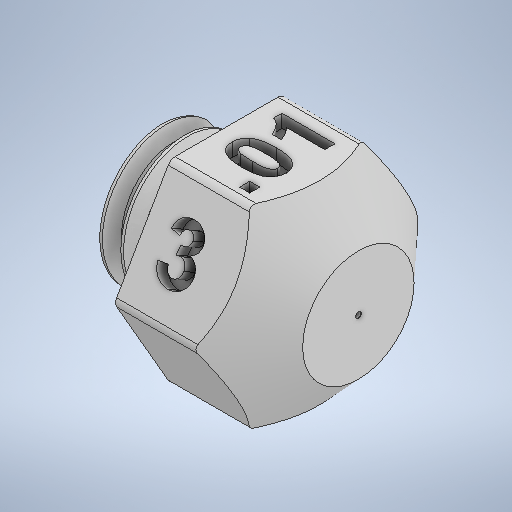
# Autodesk Inventor part: Part1
Saved by Autodesk Inventor 2025.2 (Build 292293000, 293)
## iProperties
Created: 2026-03-09
Part Number: Part1
Material: Generic
Document SubType Name: Modeling
Designer: Simon
Density: 1 g/cm^3
Appearance: Default
Author: Simon
Autodesk Inventor part; units mm, degrees
ref_plane "YZ Plane" through (0, 0, 0) normal (1, 0, 0) x (0, 1, 0)
ref_plane "XZ Plane" through (0, 0, 0) normal (0, 1, 0) x (-1, 0, 0)
ref_plane "XY Plane" through (0, 0, 0) normal (0, 0, 1) x (1, 0, 0)
sketch "Sketch1" plane through (0, 0, 0) normal (0, 0, 1) x (1, 0, 0)
  line L0 (0, 0) -> (0, 1.25)
  line L1 (0, 1.25) -> (50, 1.25)
  line L2 (0, 0) -> (0, 0.1062)
  line L3 (0, 0.1062) -> (50, 0.1062)
  line L4 (0, 0) -> (0, 0.1111)
  line L5 (0, 0.1111) -> (50, 0.1111)
  line L6 (0, 0) -> (0, 2.5)
  line L7 (0, 2.5) -> (2.5, 2.5)
  line L8 (2.5, 2.5) -> (2.5, 1.25)
  line L9 (2.5, 1.25) -> (2.5, 4.25)
  line L10 (2.5, 1.25) -> (6.7109, 1.25) construction
  line L11 (2.5, 4.25) -> (5.5, 4.25)
  line L12 (5.5, 4.25) -> (5.5, 1.25)
  line L13 (5.5, 1.25) -> (7.4811, 0.1062)
  line L14 (5.5, 1.25) -> (9.25, 1.25) construction
  line L15 (7.4811, 0.1062) -> (7.4992, 0.1111)
  line L16 (7.4811, 0.1062) -> (7.4998, 0.1062) construction
  line L17 (7.4992, 0.1111) -> (7.4992, 2.1111)
  line L18 (7.4992, 2.1111) -> (5.5, 4.25)
  line L19 (0, 0) -> (50, 0)
  dimension "d0" = 1.25
  dimension "d1" = 50
  dimension "d2" = 0.1062
  dimension "d3" = 0.1111
  dimension "d4" = 2.5
  dimension "d5" = 2.5
  dimension "d6" = 3
  dimension "d8" = 3
  dimension "d9" = 30
  dimension "d10" = 15
  dimension "d12" = 2
  dimension "d13" = 50
  constraints: 40 end point, 7 perpendicular, 7 point on line, 5 horizontal, 2 vertical, 1 equal length
  measures "d0" distance of L0.start L0.end
  measures "d1" distance of L0.end L1.end
  measures "d2" distance of L0.start L2.end
  measures "d3" distance of L0.start L4.end
  measures "d4" distance of L0.start L6.end
  measures "d5" distance of L6.end L7.end
  measures "d6" distance of L8.end L9.end
  measures "d8" distance of L9.end L11.end
  measures "d9" angle of L13 L14
  measures "d10" angle of L16 L15
  measures "d12" distance of L15.end L17.end
  measures "d13" distance of L0.start L19.end
revolve "Revolution1" add sketch "Sketch1" angle 360 about axis through (0, 0, 0) along (1, 0, 0) contours L13 L5 L15 | L6 L7 L8 L1 | L13 L1 L17 L5 | L8 L9 L11 L12 L1 | L12 L18 L17 L1
sketch "Sketch2" plane through (2.5, 0, 0) normal (-1, 0, 0) x (0, 0, 1)
  circle A0 centre (0, 0) radius 4.25 projected
  line L0 (-4.25, 0) -> (4.25, 0)
  circle A1 centre (0, 0) radius 0.1062 projected
  line L1 (4.25, 0) -> (2.125, -3.6806)
  line L2 (2.125, -3.6806) -> (-2.125, -3.6806)
  line L3 (-2.125, -3.6806) -> (-4.25, 0)
  line L4 (-4.25, 0) -> (-2.125, 3.6806)
  line L5 (-2.125, 3.6806) -> (2.125, 3.6806)
  line L6 (2.125, 3.6806) -> (4.25, 0)
  circle A2 centre (0, 0) radius 1.25
  constraints: 14 end point, 2 coincident, 2 point on circle, 1 centre point, 1 horizontal, 13 other
extrude "Extrusion1" cut sketch "Sketch2" against normal through all contours L6 A0 | A0 L1 | L5 A0 | A0 L2 | L4 A0 | A0 L3
fillet "Fillet1" radius 0.3 6 edges at (4, 3.6806, 2.125) (4, 3.6806, -2.125) (4, 0, -4.25) (4, -3.6806, -2.125) (4, -3.6806, 2.125) (4, 0, 4.25)
sketch "Sketch3" plane through (0, 0, 0) normal (0, 0, 1) x (1, 0, 0)
  line L0 (-0.35, 1.8938) -> (0.45, 1.8938)
  line L1 (-0.35, 1.8938) -> (0.05, 2.5866)
  line L2 (-0.35, 1.8938) -> (0.45, 1.8938) construction
  line L3 (0.05, 2.5866) -> (0.45, 1.8938)
  line L4 (-0.0972, 3.8266) -> (0.7028, 3.8266) construction
  line L5 (0.05, 2.5866) -> (0.05, 1.8938)
  line L6 (0.05, 1.8938) -> (0.05, 2.0671)
  line L7 (0.05, 2.0671) -> (0.45, 2.0671)
  line L8 (0.45, 2.0671) -> (-0.35, 2.0671)
  line L9 (0.05, 2.5866) -> (0.05, 2.5)
  line L10 (0.05, 2.5) -> (0.45, 2.5)
  line L11 (0.45, 2.5) -> (-0.35, 2.5)
  line L12 (-0.35, 1.8938) -> (-1.15, 1.8938)
  line L13 (0.05, 2.5866) -> (-0.75, 2.5866)
  line L14 (-0.75, 2.5866) -> (-1.15, 1.8938)
  line L15 (-0.35, 1.8938) -> (-0.75, 2.5866)
  line L16 (-0.35, 2.0671) -> (-1.15, 2.0671)
  line L17 (-0.35, 2.5) -> (-0.8, 2.5)
  line L18 (-0.75, 2.5866) -> (-0.75, 1.8938)
  line L19 (-0.35, 1.8938) -> (-0.35, 1.9938)
  circle A0 centre (-0.35, 2.0938) radius 0.1
  line L20 (-0.4077, 1.9938) -> (-0.2923, 1.9938)
  line L21 (0, 2.5) -> (2.5, 2.5) projected
  line L22 (0, 2.5) -> (-0.7, 2.5)
  line L23 (-0.7, 2.5) -> (-0.4366, 2.0438)
  line L24 (-0.4366, 2.0438) -> (-0.2634, 2.0438)
  line L25 (-0.2634, 2.0438) -> (0, 2.5)
  circle A1 centre (-0.35, 2.0938) radius 0.1
  point P0 (0, 0)
  point P1 (0, 2.5)
  dimension "d18" = 0.8
  dimension "d19" = 60
  dimension "d20" = 60
  dimension "d21" = 0.1732
  dimension "d22" = 0.0866
  dimension "d23" = 0.8
  dimension "d24" = 0.1
  dimension "d25" = 0.8
  constraints: 50 end point, 13 point on line, 7 horizontal, 4 tangent, 3 midpoint, 2 centre point, 2 equal length, 2 perpendicular, 2 point on circle, 1 coincident, 1 collinear, 1 concentric, 1 parallel, 1 vertical
  measures "d18" distance of L2.start L0.end
  measures "d19" angle of L2 L1
  measures "d20" angle of L3 L4
  measures "d21" distance of L6.start L7.start
  measures "d22" distance of L3.start L10.start
  measures "d23" distance of L2.start L12.end
  measures "d24" distance of L2.start L19.end
  measures "d25" distance between parallel lines of L5 L18
coil "Coil1" sketch "Sketch3" operation cut axis through (-10, 0, 0) along (1, 0, 0) pitch 0.8 turns 4 hand right contours A0 L24 | L24 L15 L16 L8 L1 | A0 L15 L17 L11 L1 | L8 L16 A0
extrude "Extrusion2" add sketch "Sketch2" against normal blind 3 contours L1 L2 L3 L0 A2 | L0 A2 L4 L5 L6
fillet "Fillet2" radius 0.3 6 edges at (4, 3.6806, -2.125) (4, 3.6806, 2.125) (4, 0, 4.25) (4, -3.6806, 2.125) (4, -3.6806, -2.125) (4, 0, -4.25)
sketch "Sketch4" plane through (2.5, 3.6806, 1.9518) normal (0, 1, 0) x (1, 0, 0)
  line L0 (0.6024, 0.0215) -> (0.6024, 3.9041) construction
  line L1 (0.6024, 3.9041) -> (2.6436, 3.9041) construction
  line L2 (2.6436, 3.9041) -> (2.6436, 0.0215) construction
  line L3 (2.6436, 0.0215) -> (0.6024, 0.0215) construction
  line L4 (2.6101, 0.2212) -> (2.2259, 0.2212)
  line L5 (2.2259, 0.2212) -> (2.2259, 0.6053)
  line L6 (2.2259, 0.6053) -> (2.6101, 0.6053)
  line L7 (2.6101, 0.6053) -> (2.6101, 0.2212)
  spline S0 degree 2 poles (0.6024, 1.5641) (0.6024, 1.8553) (0.8098, 2.0184) knots 0 0 0 1 1 1
  spline S1 degree 2 poles (0.8098, 2.0184) (1.0552, 2.2135) (1.6238, 2.2135) knots 0 0 0 1 1 1
  spline S2 degree 2 poles (1.6238, 2.2135) (2.1909, 2.2135) (2.4393, 2.0169) knots 0 0 0 1 1 1
  spline S3 degree 2 poles (2.4393, 2.0169) (2.6436, 1.8553) (2.6436, 1.5641) knots 0 0 0 1 1 1
  spline S4 degree 2 poles (2.6436, 1.5641) (2.6436, 1.2715) (2.1954, 0.9148) (1.6192, 0.9148) knots 0 0 0 1 2 2 2
  spline S5 degree 2 poles (1.6192, 0.9148) (1.0552, 0.9148) (0.8067, 1.1114) knots 0 0 0 1 1 1
  spline S6 degree 2 poles (0.8067, 1.1114) (0.6024, 1.273) (0.6024, 1.5641) knots 0 0 0 1 1 1
  spline S7 degree 2 poles (0.921, 1.5641) (0.921, 1.494) (1.0095, 1.3858) (1.1238, 1.3553) knots 0 0 0 1 2 2 2
  spline S8 degree 2 poles (1.1238, 1.3553) (1.2717, 1.3157) (1.6238, 1.3157) knots 0 0 0 1 1 1
  spline S9 degree 2 poles (1.6238, 1.3157) (1.9744, 1.3157) (2.2381, 1.3873) (2.325, 1.494) (2.325, 1.5641) knots 0 0 0 1 2 3 3 3
  spline S10 degree 2 poles (2.325, 1.5641) (2.325, 1.6343) (2.2366, 1.7425) (2.1223, 1.773) knots 0 0 0 1 2 2 2
  spline S11 degree 2 poles (2.1223, 1.773) (1.9744, 1.8126) (1.6238, 1.8126) knots 0 0 0 1 1 1
  spline S12 degree 2 poles (1.6238, 1.8126) (1.2717, 1.8126) (1.0095, 1.741) (0.921, 1.6343) (0.921, 1.5641) knots 0 0 0 1 2 3 3 3
  line L8 (2.6101, 3.4513) -> (2.6101, 3.0672)
  line L9 (2.6101, 3.0672) -> (1.1665, 3.0672)
  spline S13 degree 2 poles (1.1665, 3.0672) (1.3616, 2.8568) (1.4561, 2.5718) knots 0 0 0 1 1 1
  line L10 (1.4561, 2.5718) -> (1.1085, 2.5718)
  spline S14 degree 2 poles (1.1085, 2.5718) (1.0598, 2.7227) (0.7854, 3.0748) (0.6024, 3.1404) knots 0 0 0 1 2 2 2
  line L11 (0.6024, 3.1404) -> (0.6024, 3.4513)
  line L12 (0.6024, 3.4513) -> (2.6101, 3.4513)
  point P0 (-2.5, 1.9518)
  constraints: 2 other
extrude "Extrusion3" cut sketch "Sketch4" against normal blind 0.5
sketch "Sketch5" plane through (2.5, 0.15, 4.1634) normal (0, 0.5, 0.866) x (1, 0, 0)
  line L0 (0.7207, 2.9554) -> (2.413, 2.9554) construction
  line L1 (2.413, 2.9554) -> (2.413, 0.7514) construction
  line L2 (2.413, 0.7514) -> (0.7207, 0.7514) construction
  line L3 (0.7207, 0.7514) -> (0.7207, 2.9554) construction
  line L4 (0.8259, 1.4798) -> (1.1963, 1.5255)
  spline S0 degree 2 poles (1.1963, 1.5255) (1.2146, 1.3837) (1.3701, 1.2328) (1.4798, 1.2328) knots 0 0 0 1 2 2 2
  spline S1 degree 2 poles (1.4798, 1.2328) (1.5987, 1.2328) (1.7603, 1.4127) (1.7603, 1.5651) knots 0 0 0 1 2 2 2
  spline S2 degree 2 poles (1.7603, 1.5651) (1.7603, 1.71) (1.6064, 1.8792) (1.4951, 1.8792) knots 0 0 0 1 2 2 2
  spline S3 degree 2 poles (1.4951, 1.8792) (1.4219, 1.8792) (1.3198, 1.8502) knots 0 0 0 1 1 1
  line L5 (1.3198, 1.8502) -> (1.3625, 2.1627)
  spline S4 degree 2 poles (1.3625, 2.1627) (1.518, 2.1581) (1.6811, 2.3014) (1.6811, 2.4203) knots 0 0 0 1 2 2 2
  spline S5 degree 2 poles (1.6811, 2.4203) (1.6811, 2.5209) (1.5606, 2.6398) (1.4616, 2.6398) knots 0 0 0 1 2 2 2
  spline S6 degree 2 poles (1.4616, 2.6398) (1.3625, 2.6398) (1.2237, 2.5042) (1.2085, 2.3731) knots 0 0 0 1 2 2 2
  line L6 (1.2085, 2.3731) -> (0.8548, 2.4325)
  spline S7 degree 2 poles (0.8548, 2.4325) (0.8914, 2.6139) (1.0408, 2.8319) (1.3061, 2.9554) (1.4722, 2.9554) knots 0 0 0 1 2 3 3 3
  spline S8 degree 2 poles (1.4722, 2.9554) (1.7542, 2.9554) (1.925, 2.7755) knots 0 0 0 1 1 1
  spline S9 degree 2 poles (1.925, 2.7755) (2.0652, 2.6292) (2.0652, 2.4432) knots 0 0 0 1 1 1
  spline S10 degree 2 poles (2.0652, 2.4432) (2.0652, 2.181) (1.7771, 2.024) knots 0 0 0 1 1 1
  spline S11 degree 2 poles (1.7771, 2.024) (1.9494, 1.9874) (2.1536, 1.7298) (2.1536, 1.5484) knots 0 0 0 1 2 2 2
  spline S12 degree 2 poles (2.1536, 1.5484) (2.1536, 1.2847) (1.7695, 0.9142) (1.4829, 0.9142) knots 0 0 0 1 2 2 2
  spline S13 degree 2 poles (1.4829, 0.9142) (1.2116, 0.9142) (0.8548, 1.2267) (0.8259, 1.4798) knots 0 0 0 1 2 2 2
  point P0 (-2.5, 1.9518)
  constraints: 2 other
extrude "Extrusion4" cut sketch "Sketch5" against normal blind 0.5
body "Solid1"
